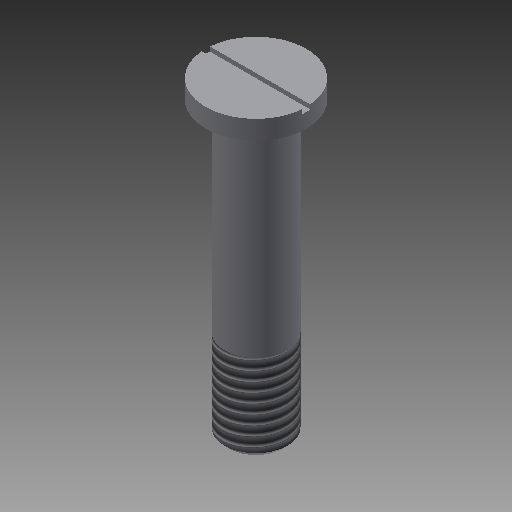
# Autodesk Inventor part: May Tec 1.63.14041/3_Clamping stud 40x40
Saved by Autodesk Inventor 2018 (Build 220112000, 112)
## iProperties
Category: PARTsolutions
Company: MAYTEC
Created: 2012-12-11
Part Number: May Tec 1.63.14041/3_Clamping stud 40x40
Catalog Web Link: www.cadenas.de
Description: 1.63.1x-Clamp bolt with thread
Vendor: MAYTEC
Document SubType Name: Modeling
Designer: PARTuser1
Manufacturer: MAYTEC
Density: 1 g/cm^3
Material: Generic
Appearance: RGB(192.00000375509219,192.00000375509219,192.00000375509219)
PSOL_IDENT_0: {\\10.0.0.242\data_v9\23d-libs\maytec\maytec_3d\anbauzubehoer\gelenke\gelenke_pg_30-50_spannhebel\sp
PSOL_IDENT_1: annbolzen_mit_gewinde.prj},223 {VTYP=3D},{NB=May Tec 1.63.14041/3_Clamping stud 40x40},{LINA=May Tec
PSOL_IDENT_2: 1.63.14041/3_Clamping stud 40x40},{NN=1.63.1x},{DATE=14.09.2010 08:31:40},{GEOMDATE=15.02.2008 00:0
PSOL_IDENT_3: 0:00},{VERSION=},{LINEID=30},{LINESUBID=-1},{WBVAR=}  {NB=May Tec 1.63.14041/3_Clamping stud 40x40},
PSOL_IDENT_4: {LINA=May Tec 1.63.14041/3_Clamping stud 40x40},{KT=DUMMY},{IDNR=},{PARTNR=1.63.14041/3},{GELENKNR=1
PSOL_IDENT_5: .63.14041},{DESCRIPTION=Spannbolzen fuer Gelenk 40x40},{L=49.0},{D=10.0},{DK=16.0},{HK=3.0},{GEWINDE
PSOL_IDENT_6: =10.000},{GL=14.0},{XTRANS=Clamping stud 40x40}
CNS_NT: Clamp bolt with thread
CNS_NB: May Tec 1.63.14041/3_Clamping stud 40x40
CNS_NBSYN: May Tec $PARTNR._$XTRANS.
CNS_LINA: May Tec 1.63.14041/3_Clamping stud 40x40
CNS_PARTNR: 1.63.14041/3
CNS_GELENKNR: 1.63.14041
CNS_DESCRIPTION: Clamping stud 40x40
CNS_L: 49.0
CNS_D: 10.0
CNS_DK: 16.0
CNS_HK: 3.0
CNS_GEWINDE: 10.000
CNS_GL: 14.0
CNS_XTRANS: Clamping stud 40x40
SUPPLIER: MAYTEC
ARTICLENO: May Tec 1.63.14041/3_Clamping stud 40x40
BOMINFO: May Tec 1.63.14041/3_Clamping stud 40x40
CREATOR: CADENAS GmbH
Title: May Tec 1.63.14041/3_Clamping stud 40x40
Author: Cadenas PARTsolutions
Comments: Clamp bolt with thread
Autodesk Inventor part; units mm, degrees
sketch "Skizze_1" plane through (0, 21.5, 0) normal (0, 1, 0) x (1, 0, 0)
  circle A0 centre (0, 0) radius 8
  constraints: 1 centre point
extrude "Extrusion1" add sketch "Skizze_1" along normal blind 3
sketch "Skizze_3" plane through (0, 0, 0) normal (0, 0, 1) x (1, 0, 0)
  line L0 (-8, 24.5) -> (-8, 23.8)
  line L1 (-8, 23.8) -> (8, 23.8)
  line L2 (8, 23.8) -> (8, 24.5)
  line L3 (8, 24.5) -> (-8, 24.5)
  constraints: 8 end point
extrude "Extrusion2" cut sketch "Skizze_3" along normal mid plane 1.3
sketch "Skizze_2" plane through (0, 0, 0) normal (0, 0, 1) x (1, 0, 0)
  line L0 (0, -24.5) -> (0, 21.5)
  line L1 (0, 21.5) -> (5, 21.5)
  line L2 (5, 21.5) -> (5, -23.58)
  line L3 (5, -23.58) -> (4.08, -24.5)
  line L4 (4.08, -24.5) -> (0, -24.5)
  line L5 (0, -24.5) -> (0, 21.5)
  constraints: 12 end point
revolve "Revolution1" add sketch "Skizze_2" angle 360 about axis through (0, -24.5, 0) along (0, -1, 0)
thread "Thread1" size "M10x1.5" class "6g" standard "ISO Metric profile" length 14 offset 32
ref_plane "hebel_XY" through (0, 24.5, 0) normal (0, 1, 0) x (-1, 0, 0)
ref_plane "hebel_YZ" through (0, 24.5, 0) normal (-1, 0, 0) x (0, 0, 1)
ref_plane "hebel_ZX" through (0, 24.5, 0) normal (0, 0, 1) x (0, 1, 0)
body "Solid1"
